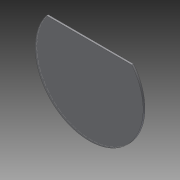
# Autodesk Inventor part: Top Plate
Saved by Autodesk Inventor 2015 (Build 190159000, 159)
## iProperties
Created: 2014-11-13
Part Number: Top Plate
Material: Generic
Document SubType Name: Modeling
Designer: karl
Density: 1 g/cm^3
Appearance: Default
Author: karl
Autodesk Inventor part; units mm, degrees
ref_plane "YZ Plane" through (0, 0, 0) normal (1, 0, 0) x (0, 1, 0)
ref_plane "XZ Plane" through (0, 0, 0) normal (0, 1, 0) x (-1, 0, 0)
ref_plane "XY Plane" through (0, 0, 0) normal (0, 0, 1) x (1, 0, 0)
sketch "Sketch1" plane through (0, 0, 0) normal (0, 1, 0) x (-1, 0, 0)
  circle A0 centre (0, 0) radius 90
  line L0 (-71.239, 55) -> (71.239, 55)
  dimension "d0" = 180
  dimension "d1" = 55
  constraints: 2 end point, 2 point on circle, 1 centre point, 1 coincident, 1 horizontal
  measures "d0" diameter of A0
  measures "d1" distance from line of point (0, 0) L0
extrude "Extrusion1" add sketch "Sketch1" along normal blind 3 contours A0 L0 picked at (-1.0947, 6.6866)
sketch "Sketch2" plane through (0, 3, 0) normal (0, 1, 0) x (1, 0, 0)
  line L0 (-71.239, -55) -> (71.239, -55) projected
  line L1 (-70, -55) -> (-60, -55)
  line L2 (-60, -55) -> (-60, -52)
  line L3 (-60, -52) -> (-70, -52)
  line L4 (-70, -52) -> (-70, -55)
  line L5 (-30, -55) -> (-10, -55)
  line L6 (-10, -55) -> (-10, -52)
  line L7 (-10, -52) -> (-30, -52)
  line L8 (-30, -52) -> (-30, -55)
  point P0 (0, 0)
  dimension "d4" = 10
  dimension "d5" = 3
  dimension "d6" = 20
  dimension "d7" = 3
  dimension "d8" = 10
  dimension "d9" = 30
  constraints: 16 end point, 4 parallel, 2 horizontal, 2 perpendicular, 2 point on line
  measures "d4" distance of L3.end L2.end
  measures "d5" distance of L2.end L1.end
  measures "d6" distance of L7.end L6.end
  measures "d7" distance of L6.end L5.end
  measures "d8" distance from line of point (0, 0) L6
  measures "d9" distance between parallel lines of L2 L8
extrude "Extrusion2" cut sketch "Sketch2" against normal blind 3
sketch "Sketch3" plane through (0, 3, 0) normal (0, 1, 0) x (1, 0, 0)
  line L0 (-57, -42) -> (-60, -42)
  line L1 (-60, -42) -> (-60, -22)
  line L2 (-60, -22) -> (-57, -22)
  line L3 (-57, -22) -> (-57, -42)
  line L4 (-57, -12) -> (-60, -12)
  line L5 (-60, -12) -> (-60, -2)
  line L6 (-60, -2) -> (-57, -2)
  line L7 (-57, -2) -> (-57, -12)
  line L8 (-57, 18) -> (-60, 18)
  line L9 (-60, 18) -> (-60, 38)
  line L10 (-60, 38) -> (-57, 38)
  line L11 (-57, 38) -> (-57, 18)
  line L12 (-70, -52) -> (-60, -52) projected
  point P0 (0, 0)
  dimension "d12" = 3
  dimension "d13" = 20
  dimension "d14" = 3
  dimension "d15" = 10
  dimension "d16" = 3
  dimension "d17" = 20
  dimension "d18" = 10
  dimension "d19" = 10
  dimension "d20" = 20
  dimension "d21" = 57
  constraints: 24 end point, 6 parallel, 3 horizontal, 3 perpendicular, 1 collinear, 1 point on line
  measures "d12" distance of L1.end L2.end
  measures "d13" distance of L0.end L1.end
  measures "d14" distance of L5.end L6.end
  measures "d15" distance of L4.end L5.end
  measures "d16" distance of L9.end L10.end
  measures "d17" distance of L8.end L9.end
  measures "d18" distance between parallel lines of L12 L0
  measures "d19" distance between parallel lines of L4 L2
  measures "d20" distance between parallel lines of L8 L6
  measures "d21" distance from line of point (0, 0) L11
extrude "Extrusion3" cut sketch "Sketch3" against normal blind 3
sketch "Sketch4" plane through (0, 3, 0) normal (0, 1, 0) x (1, 0, 0)
  line L0 (-42.5, -34) -> (-52.5, -34)
  line L1 (-52.5, -34) -> (-52.5, -37)
  line L2 (-52.5, -37) -> (-42.5, -37)
  line L3 (-42.5, -37) -> (-42.5, -34)
  line L4 (-42.5, 14) -> (-52.5, 14)
  line L5 (-52.5, 14) -> (-52.5, 11)
  line L6 (-52.5, 11) -> (-42.5, 11)
  line L7 (-42.5, 11) -> (-42.5, 14)
  line L8 (-70, -52) -> (-60, -52) projected
  line L9 (-57, -22) -> (-57, -42) projected
  point P0 (0, 0)
  dimension "d24" = 10
  dimension "d25" = 3
  dimension "d26" = 10
  dimension "d27" = 3
  dimension "d28" = 15
  dimension "d29" = 45
  dimension "d30" = 4.5
  constraints: 16 end point, 4 parallel, 2 horizontal, 2 perpendicular, 1 point on line
  measures "d24" distance of L2.end L1.end
  measures "d25" distance of L1.end L0.end
  measures "d26" distance of L6.end L5.end
  measures "d27" distance of L5.end L4.end
  measures "d28" distance between parallel lines of L2 L8
  measures "d29" distance between parallel lines of L0 L6
  measures "d30" distance between parallel lines of L9 L1
extrude "Extrusion4" cut sketch "Sketch4" against normal blind 3
mirror "Mirror1" about plane through (0, 0, 0) normal (1, 0, 0) of "Extrusion4", "Extrusion3", "Extrusion2"
body "Solid1"
